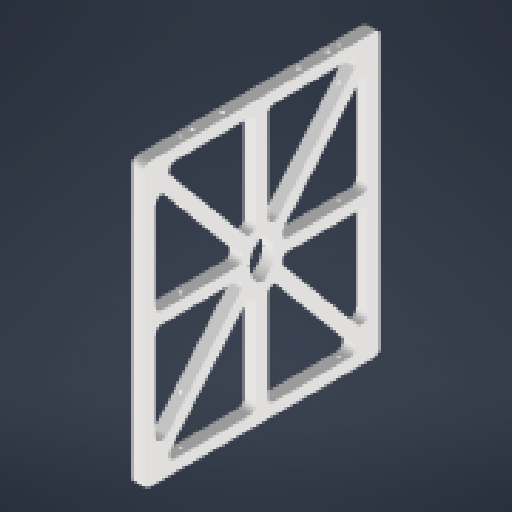
# Autodesk Inventor part: Halterung_Aufbau
Saved by Autodesk Inventor 2027 (Build 310192060, 192F)
## iProperties
Created: 2026-07-21
Part Number: Halterung_Aufbau
Material: Generic
Document SubType Name: Modeling
Designer: kw
Density: 1 g/cm^3
Appearance: Default
Author: kw
Autodesk Inventor part; units mm, degrees
ref_plane "YZ Plane" through (0, 0, 0) normal (1, 0, 0) x (0, 1, 0)
ref_plane "XZ Plane" through (0, 0, 0) normal (0, 1, 0) x (-1, 0, 0)
ref_plane "XY Plane" through (0, 0, 0) normal (0, 0, 1) x (1, 0, 0)
sketch "Sketch1" plane through (0, 0, 0) normal (0, 1, 0) x (-1, 0, 0)
  line L0 (0, 0) -> (389, 0)
  line L1 (389, 0) -> (389, -464)
  line L2 (389, -464) -> (0, -464)
  line L3 (0, -464) -> (0, 0)
  line L4 (369, -444) -> (369, -20)
  line L5 (369, -20) -> (20, -20)
  line L6 (20, -20) -> (20, -444)
  line L7 (20, -444) -> (369, -444)
  line L8 (184.5, 0) -> (204.5, 0)
  line L9 (204.5, 0) -> (204.5, -464)
  line L10 (204.5, -464) -> (184.5, -464)
  line L11 (184.5, -464) -> (184.5, 0)
  line L12 (0, -222) -> (389, -222)
  line L13 (389, -222) -> (389, -242)
  line L14 (389, -242) -> (0, -242)
  line L15 (0, -242) -> (0, -222)
  line L16 (396.6632, -6.4246) -> (7.6632, -470.4246)
  line L17 (381.3368, 6.4246) -> (-7.6632, -457.5754)
  line L18 (7.6632, 6.4246) -> (396.6632, -457.5754)
  line L19 (-7.6632, -6.4246) -> (381.3368, -470.4246)
  point P0 (369, -222)
  point P1 (215.933, -222)
  point P2 (369, -39.4213)
  point P3 (369, -242)
  point P4 (369, -424.5787)
  point P5 (215.933, -242)
  point P6 (184.5, -20)
  point P7 (184.5, -204.5067)
  point P8 (29.8166, -20)
  point P9 (20, -424.5787)
  point P10 (20, -242)
  point P11 (173.067, -242)
  point P12 (204.5, -259.4933)
  point P13 (359.1834, -444)
  point P14 (204.5, -444)
  point P15 (20, -39.4213)
  point P16 (173.067, -222)
  point P17 (20, -222)
  point P18 (359.1834, -20)
  point P19 (204.5, -204.5067)
  point P20 (204.5, -20)
  point P21 (184.5, -444)
  point P22 (29.8166, -444)
  point P23 (184.5, -259.4933)
  dimension "d0" = 389
  dimension "d1" = 464
  dimension "d2" = 20
  dimension "d3" = 20
  dimension "d4" = 20
  constraints: 40 end point, 8 parallel, 4 perpendicular, 4 point on line, 3 horizontal, 3 other
  measures "d0" distance of L1.end L2.end
  measures "d1" distance of L0.end L1.end
  measures "d2" distance between parallel lines of L1 L4
  measures "d3" distance of L9.end L10.end
  measures "d4" distance of L12.end L13.end
extrude "Extrusion1" add sketch "Sketch1" along normal blind 20 contours L11 L5 L18 L0 | L0 L9 L5 L11 | L0 L17 L5 L9 | L18 L5 L6 L19 L3 L0 | L5 L9 L17 L18 L11 | L0 L1 L16 L4 L5 L17 | L18 L11 L12 L19 L6 L5 | L18 L17 L12 L11 | L5 L4 L16 L12 L9 L17 | L9 L12 L18 L17 | L19 L6 L12 L3 | L12 L17 L11 | L11 L17 L19 L12 | L18 L12 L17 | L1 L12 L4 L16 | L12 L16 L18 L9 | L9 L18 L12 | L12 L6 L14 L3 | L17 L12 L18 L9 L16 L14 L19 L11 | L11 L19 L17 | L19 L17 L14 L6 L12 | L1 L14 L4 L12 | L18 L16 L9 | L12 L4 L14 L18 L16 | L14 L6 L17 L3 | L19 L14 L11 | L11 L14 L17 L19 | L1 L18 L4 L14 | L16 L18 L14 L9 | L9 L14 L16 | L17 L6 L7 L16 L2 L3 | L14 L19 L16 L11 | L11 L16 L7 L6 L17 L14 | L14 L16 L19 | L1 L2 L19 L7 L4 L18 | L14 L18 L4 L7 L19 L9 | L9 L19 L16 L14 | L16 L19 L9 L7 L11 | L16 L7 L11 L2 | L7 L9 L2 L11 | L2 L9 L7 L19
fillet "Fillet1" radius 10 28 edges at (-389, 10, 0) (0, 10, 0) (0, 10, -464) (-389, 10, -464) (-369, 10, -424.5787) (-359.1834, 10, -444) (-369, 10, -242) (-369, 10, -222) (-204.5, 10, -444) (-204.5, 10, -259.4933) (-215.933, 10, -242) (-215.933, 10, -222) (-204.5, 10, -204.5067) (-184.5, 10, -204.5067) (-173.067, 10, -222) (-173.067, 10, -242) (-184.5, 10, -259.4933) (-369, 10, -39.4213) (-359.1834, 10, -20) (-204.5, 10, -20) (-184.5, 10, -20) (-29.8166, 10, -20) (-20, 10, -39.4213) (-20, 10, -222) (-20, 10, -242) (-20, 10, -424.5787) (-29.8166, 10, -444) (-184.5, 10, -444)
sketch "Sketch2" plane through (0, 20, 0) normal (0, 1, 0) x (1, 0, 0)
  line L0 (-389, 454) -> (-389, 10) projected
  line L1 (-389, 232) -> (0, 232)
  line L2 (0, 10) -> (0, 454) projected
  line L3 (-379, 0) -> (-10, 0) projected
  line L4 (-194.5, 0) -> (-194.5, 464)
  line L5 (-10, 464) -> (-379, 464) projected
  arc A0 (-194.5, 265) -> (-194.5, 199) centre (-177.7668, 232) ccw
  arc A1 (-194.5, 199) -> (-194.5, 265) centre (-211.2332, 232) ccw
  point P0 (0, 0)
  dimension "d12" = 66
  dimension "d13" = 37
  dimension "d14" = 37
  constraints: 4 end point, 4 midpoint, 4 point on circle, 2 centre point, 2 point on line
  measures "d12" distance of A0.start A0.end
  measures "d13" radius of A0
  measures "d14" radius of A1
extrude "Extrusion2" cut sketch "Sketch2" against normal through all
fillet "Fillet2" radius 10 2 edges at (-194.5, 10, -265) (-194.5, 10, -199)
sketch "Sketch6" plane through (-10, 0, -464) normal (0, 0, -1) x (-1, 0, 0)
  line L0 (369, 20) -> (369, 0) projected
  line L1 (0, 20) -> (369, 20) projected
  line L2 (0, 0) -> (0, 20) projected
  line L3 (0, 0) -> (369, 0) projected
  line L4 (0, 10) -> (80, 10)
  line L5 (0, 10) -> (80, 10) construction
  line L6 (80, 10) -> (129, 10)
  line L7 (369, 10) -> (303.0267, 10)
  line L8 (369, 10) -> (434.9733, 10) construction
  line L9 (303.0267, 10) -> (254.0267, 10)
  dimension "d48" = 80
  dimension "d49" = 0
  dimension "d50" = 49
  dimension "d51" = 180
  dimension "d52" = 180
  dimension "d53" = 49
  dimension "d54" = 180
  constraints: 12 end point, 4 collinear, 3 horizontal, 2 midpoint
  measures "d48" distance of L4.start L4.end
  measures "d49" distance between parallel lines of L4 L5
  measures "d50" distance of L4.end L6.end
  measures "d51" angle of L6 L4
  measures "d52" angle of L7 L8
  measures "d53" distance of L7.end L9.end
  measures "d54" angle of L9 L7
hole "Hole2" at (-90, 10, -464) at (-139, 10, -464) at (-264.0267, 10, -464) at (-313.0267, 10, -464) direction (0, 0, 1) diameter 4.917 depth 20 thread size "M6x1" class "6H" standard "ISO Metric profile"
sketch "Sketch8" plane through (-379, 0, 0) normal (0, 0, 1) x (1, 0, 0)
  line L0 (379, 0) -> (379, 20) projected
  line L1 (369, 20) -> (369, 0) projected
  line L2 (0, 20) -> (369, 20) projected
  line L3 (0, 0) -> (0, 20) projected
  line L4 (0, 0) -> (369, 0) projected
  line L5 (0, 10) -> (369, 10)
  line L6 (178.3025, 0) -> (178.3025, 20) projected
  line L7 (178.3025, 10) -> (308.3025, 10)
  line L8 (308.3025, 10) -> (48.3025, 10)
  dimension "d46" = 130
  dimension "d47" = 260
  constraints: 6 end point, 3 midpoint, 2 coincident, 2 point on line
  measures "d46" distance of L7.start L7.end
  measures "d47" distance of L7.end L8.end
hole "Hole3" at (-330.6975, 10, 0) at (-70.6975, 10, 0) direction (0, 0, -1) diameter 4.917 depth 20 thread size "M6x1" class "6H" standard "ISO Metric profile"
body "Solid1"
